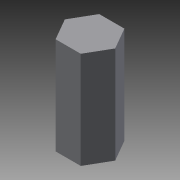
# Autodesk Inventor part: koara_march
Saved by Autodesk Inventor 2015 (Build 190159000, 159)
## iProperties
Created: 2016-08-19
Part Number: koara_march
Material: 一般
Document SubType Name: Modeling
Designer: Ryo
Density: 1 g/cm^3
Appearance: 既定
Mass: 429.657 g
Surface Area: 347.153 cm^2
Volume: 429.657 cm^3
Author: Ryo
Autodesk Inventor part; units mm, degrees
ref_plane "YZ Plane" through (0, 0, 0) normal (1, 0, 0) x (0, 1, 0)
ref_plane "XZ Plane" through (0, 0, 0) normal (0, 1, 0) x (-1, 0, 0)
ref_plane "XY Plane" through (0, 0, 0) normal (0, 0, 1) x (1, 0, 0)
sketch "スケッチ1" plane through (0, 0, 0) normal (0, 0, 1) x (1, 0, 0)
  line L0 (35, 0) -> (17.5, -30.3109)
  line L1 (17.5, -30.3109) -> (-17.5, -30.3109)
  line L2 (-17.5, -30.3109) -> (-35, 0)
  line L3 (-35, 0) -> (-17.5, 30.3109)
  line L4 (-17.5, 30.3109) -> (17.5, 30.3109)
  line L5 (17.5, 30.3109) -> (35, 0)
  point P0 (0, 0)
  point P1 (0, 0)
  dimension "d0" = 35
  constraints: 12 end point, 1 coincident, 13 other
  measures "d0" distance of L4.end L3.end
extrude "押し出し1" add sketch "スケッチ1" along normal blind 135
